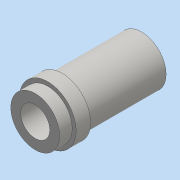
# Autodesk Inventor part: Objective-Lens
Saved by Autodesk Inventor 2016 SP1 (Build 200210100, 210)
## iProperties
Created: 2016-03-24
Part Number: Objective-Lens
Material: Generic
Document SubType Name: Modeling
Designer: Mohamed A.
Density: 1 g/cm^3
Appearance: Default
Author: Mohamed A.
Autodesk Inventor part; units mm, degrees
ref_plane "XZ Plane" through (0, 0, 0) normal (0, 1, 0) x (-1, 0, 0)
sketch "Sketch1" plane through (0, 0, 0) normal (0, 0, 1) x (1, 0, 0)
  line L0 (6.05, 0) -> (6.05, 41.3489)
  line L1 (6.05, 0) -> (10.15, 0)
  line L2 (10.15, 0) -> (10.15, 5.2)
  line L3 (10.15, 5.2) -> (11.8, 5.2)
  line L4 (11.8, 5.2) -> (11.8, 11.2)
  line L5 (11.8, 11.2) -> (10.15, 11.2)
  line L6 (0, -9.1) -> (0, 54.6) construction
  line L7 (10.15, 11.2) -> (10.15, 44.2)
  line L8 (6.25, 45.5) -> (10.15, 44.2)
  line L9 (6.25, 45.5) -> (3.75, 45.5)
  line L10 (3.75, 45.5) -> (3.75, 41.3489)
  line L11 (3.75, 41.3489) -> (6.05, 41.3489)
  point P0 (0, 0)
  dimension "d0" = 10.15
  dimension "d1" = 4.1
  dimension "d2" = 11.2
  dimension "d3" = 11.8
  dimension "d5" = 6.05
  dimension "d9" = 44.2
  dimension "d11" = 45.5
  dimension "d13" = 6
  dimension "d14" = 3.75
  dimension "d15" = 4.1511
  dimension "d16" = 6.25
  constraints: 22 end point, 4 perpendicular, 3 horizontal, 3 vertical, 1 collinear
  measures "d0" distance of point (0, 0) L1.end
  measures "d1" distance between parallel lines of L0 L2
  measures "d2" distance from line of point (0, 0) L5
  measures "d3" distance from line of point (0, 0) L4
  measures "d5" distance from line of point (0, 0) L0
  measures "d9" vertical distance of point (0, 0) L7.end
  measures "d11" vertical distance of point (0, 0) L8.start
  measures "d13" distance between parallel lines of L3 L5
  measures "d14" distance from line of L6 L9.end
  measures "d15" distance between parallel lines of L11 L9
  measures "d16" distance from line of L6 L8.start
revolve "Revolution1" add sketch "Sketch1" angle 360 about axis through (0, -10, 0) along (0, 1, 0)
body "Solid1"
